Autodesk Inventor part; units mm, degrees
(part 2 of 2)
  arc A179 (-8.5428, 20.014) -> (-8.1409, 20.1954) centre (-9.6846, 23.0787) ccw
  arc A180 (-9.5743, 19.8012) -> (-8.5428, 20.014) centre (-9.7473, 23.247) ccw
  arc A181 (-10.6109, 19.9132) -> (-9.5743, 19.8012) centre (-9.7407, 23.1144) ccw
  arc A182 (-11.5656, 20.3424) -> (-10.6109, 19.9132) centre (-9.7333, 23.1418) ccw
  arc A183 (-12.3588, 21.0513) -> (-11.5656, 20.3424) centre (-9.6135, 23.3247) ccw
  line L45 (-12.3588, 21.0513) -> (-12.436, 21.1445)
  line L46 (-12.436, 21.1445) -> (-12.8142, 20.787)
  line L47 (-12.8142, 20.787) -> (-13.1923, 20.4294)
  line L48 (-13.1923, 20.4294) -> (-13.1528, 20.3728)
  arc A184 (-13.1528, 20.3728) -> (-13.1252, 20.3384) centre (-12.8824, 20.5615) ccw
  arc A185 (-13.1252, 20.3384) -> (-13.0498, 20.2573) centre (-6.3279, 26.584) ccw
  arc A186 (-13.0498, 20.2573) -> (-12.9584, 20.1617) centre (-6.8687, 26.075) ccw
  arc A187 (-12.9584, 20.1617) -> (-12.8577, 20.0592) centre (-4.4477, 28.4259) ccw
  arc A188 (-12.8577, 20.0592) -> (-12.5717, 19.7931) centre (-9.2726, 23.6258) ccw
  arc A189 (-12.5717, 19.7931) -> (-12.2821, 19.5663) centre (-9.9736, 22.8114) ccw
  arc A190 (-12.2821, 19.5663) -> (-11.9733, 19.3675) centre (-9.9819, 22.7997) ccw
  arc A191 (-11.9733, 19.3675) -> (-11.6297, 19.1857) centre (-9.4749, 23.6737) ccw
  arc A192 (-11.6297, 19.1857) -> (-11.2883, 19.0399) centre (-9.8103, 22.9749) ccw
  arc A193 (-11.2883, 19.0399) -> (-10.9284, 18.9216) centre (-9.686, 23.306) ccw
  arc A194 (-10.9284, 18.9216) -> (-10.5594, 18.8334) centre (-9.6828, 23.3174) ccw
  arc A195 (-10.5594, 18.8334) -> (-10.1908, 18.7779) centre (-9.742, 23.0144) ccw
  arc A196 (-10.1908, 18.7779) -> (-9.9934, 18.7649) centre (-9.929, 21.2498) ccw
  arc A197 (-9.9934, 18.7649) -> (-9.7075, 18.7614) centre (-9.7234, 29.1694) ccw
  arc A198 (-9.7075, 18.7614) -> (-9.4242, 18.7657) centre (-9.7237, 29.3221) ccw
  arc A199 (-9.4242, 18.7657) -> (-9.2413, 18.7794) centre (-9.4803, 20.7415) ccw
  arc A200 (-9.5434, 20.4503) -> (-9.0552, 20.5352) centre (-9.8712, 23.7792) ccw
  arc A201 (-9.0552, 20.5352) -> (-8.6122, 20.6889) centre (-9.7096, 23.1369) ccw
  arc A202 (-8.6122, 20.6889) -> (-8.2116, 20.9135) centre (-9.6623, 23.0313) ccw
  arc A203 (-8.2116, 20.9135) -> (-7.8493, 21.2097) centre (-9.7746, 23.1952) ccw
  arc A204 (-7.8493, 21.2097) -> (-7.7329, 21.3272) centre (-10.6671, 24.1156) ccw
  arc A205 (-7.7329, 21.3272) -> (-7.622, 21.4489) centre (-10.618, 24.069) ccw
  arc A206 (-7.622, 21.4489) -> (-7.5253, 21.5617) centre (-13.3375, 26.4473) ccw
  arc A207 (-7.5253, 21.5617) -> (-7.5138, 21.5934) centre (-7.563, 21.5934) ccw
  arc A208 (-7.5138, 21.5934) -> (-7.5197, 21.607) centre (-7.5325, 21.5934) ccw
  arc A209 (-7.5197, 21.607) -> (-7.884, 21.95) centre (-910.3811, -936.9121) ccw
  arc A210 (-7.884, 21.95) -> (-8.2435, 22.2882) centre (-469.987, -469.0133) ccw
  arc A211 (-8.2435, 22.2882) -> (-8.2689, 22.3041) centre (-8.2969, 22.2313) ccw
  arc A212 (-8.2689, 22.3041) -> (-8.2777, 22.3021) centre (-8.2718, 22.2966) ccw
  arc A213 (-8.2777, 22.3021) -> (-8.3041, 22.2731) centre (-7.5009, 21.5676) ccw
  arc A214 (-8.3041, 22.2731) -> (-8.3348, 22.236) centre (-7.7116, 21.7527) ccw
  arc A215 (-8.3348, 22.236) -> (-8.3684, 22.1908) centre (-7.1758, 21.3372) ccw
  arc A216 (-8.5704, 21.9586) -> (-8.3684, 22.1908) centre (-9.6953, 23.1405) ccw
  arc A217 (-8.8146, 21.7653) -> (-8.5704, 21.9586) centre (-9.7506, 23.1987) ccw
  arc A218 (-9.0914, 21.6184) -> (-8.8146, 21.7653) centre (-9.7618, 23.2158) ccw
  arc A219 (-9.3897, 21.524) -> (-9.0914, 21.6184) centre (-9.7586, 23.2082) ccw
  arc A220 (-9.5647, 21.5009) -> (-9.3897, 21.524) centre (-9.6138, 22.5471) ccw
  arc A221 (-9.7914, 21.4994) -> (-9.5647, 21.5009) centre (-9.6959, 24.2957) ccw
  arc A222 (-10.0176, 21.5163) -> (-9.7914, 21.4994) centre (-9.6958, 24.2978) ccw
  arc A223 (-10.1914, 21.5513) -> (-10.0176, 21.5163) centre (-9.8956, 22.5709) ccw
  arc A224 (-10.4567, 21.6554) -> (-10.1914, 21.5513) centre (-9.7563, 23.051) ccw
  arc A225 (-10.7116, 21.8099) -> (-10.4567, 21.6554) centre (-9.618, 23.3266) ccw
  arc A226 (-10.938, 22.0024) -> (-10.7116, 21.8099) centre (-9.6252, 23.3166) ccw
  arc A227 (-11.1179, 22.2194) -> (-10.938, 22.0024) centre (-9.8722, 23.0693) ccw
  arc A228 (-11.1179, 22.2194) -> (-11.1427, 22.2537) centre (-11.7714, 21.7735) ccw
  arc A229 (-11.1427, 22.2537) -> (-11.1661, 22.2818) centre (-11.4888, 21.9894) ccw
  arc A230 (-11.1661, 22.2818) -> (-11.1862, 22.3026) centre (-11.4945, 21.9842) ccw
  arc A231 (-11.1862, 22.3026) -> (-11.1949, 22.3043) centre (-11.1919, 22.2966) ccw
  arc A232 (-11.1949, 22.3043) -> (-11.2195, 22.289) centre (-11.1681, 22.2342) ccw
  arc A233 (-11.2195, 22.289) -> (-11.5799, 21.9506) centre (486.2167, -507.9155) ccw
  arc A234 (-11.5799, 21.9506) -> (-11.945, 21.6075) centre (951.9894, -1003.6952) ccw
  arc A235 (-11.945, 21.6075) -> (-11.9507, 21.5943) centre (-11.9326, 21.5943) ccw
  arc A236 (-11.9507, 21.5943) -> (-11.9489, 21.5889) centre (-11.9416, 21.5943) ccw
  arc A237 (-11.9489, 21.5889) -> (-11.923, 21.5541) centre (-5.8217, 26.1081) ccw
  arc A238 (-11.923, 21.5541) -> (-11.8927, 21.5141) centre (-9.796, 23.1417) ccw
  arc A239 (-11.8927, 21.5141) -> (-11.8566, 21.4683) centre (-8.0644, 24.4859) ccw
  arc A240 (-11.8566, 21.4683) -> (-11.6693, 21.2609) centre (-10.1114, 22.857) ccw
  arc A241 (-11.6693, 21.2609) -> (-11.4378, 21.0549) centre (-9.3184, 23.6694) ccw
  arc A242 (-11.4378, 21.0549) -> (-11.1876, 20.8706) centre (-9.3086, 23.6815) ccw
  arc A243 (-11.1876, 20.8706) -> (-10.944, 20.7285) centre (-9.9098, 22.7821) ccw
  arc A244 (-10.944, 20.7285) -> (-10.7872, 20.6592) centre (-10.181, 22.2437) ccw
  arc A245 (-10.7872, 20.6592) -> (-10.5834, 20.5871) centre (-9.2725, 24.618) ccw
  arc A246 (-10.5834, 20.5871) -> (-10.3752, 20.5253) centre (-9.2666, 24.6361) ccw
  arc A247 (-10.3752, 20.5253) -> (-10.2042, 20.4879) centre (-9.9036, 22.274) ccw
  arc A248 (-10.2042, 20.4879) -> (-10.0507, 20.4678) centre (-9.8539, 22.569) ccw
  arc A249 (-10.0507, 20.4678) -> (-9.8548, 20.4531) centre (-9.5485, 25.8313) ccw
  arc A250 (-9.8548, 20.4531) -> (-9.6658, 20.4456) centre (-9.5457, 25.8799) ccw
  arc A251 (-9.6658, 20.4456) -> (-9.5434, 20.4503) centre (-9.6433, 21.4646) ccw
  arc A252 (-9.5151, 22.1652) -> (-9.26, 22.2834) centre (-9.7491, 23.0046) ccw
  arc A253 (-9.26, 22.2834) -> (-9.0536, 22.4774) centre (-9.7633, 23.0256) ccw
  arc A254 (-9.0536, 22.4774) -> (-8.9194, 22.7243) centre (-9.7513, 23.0163) ccw
  arc A255 (-8.9194, 22.7243) -> (-8.8734, 22.9959) centre (-9.6884, 22.9943) ccw
  arc A256 (-8.8734, 22.9959) -> (-8.9614, 23.3705) centre (-9.7212, 22.9942) ccw
  arc A257 (-8.9614, 23.3705) -> (-9.2064, 23.6715) centre (-9.7465, 22.9817) ccw
  arc A258 (-9.2064, 23.6715) -> (-9.5559, 23.8357) centre (-9.7402, 22.9898) ccw
  arc A259 (-9.5559, 23.8357) -> (-9.9363, 23.8281) centre (-9.73, 23.0363) ccw
  arc A260 (-9.9363, 23.8281) -> (-10.1561, 23.7402) centre (-9.6975, 22.9113) ccw
  arc A261 (-10.1561, 23.7402) -> (-10.3382, 23.6031) centre (-9.7607, 23.0257) ccw
  arc A262 (-10.3382, 23.6031) -> (-10.4753, 23.421) centre (-9.7607, 23.0257) ccw
  arc A263 (-10.4753, 23.421) -> (-10.5631, 23.2012) centre (-9.6464, 22.9624) ccw
  arc A264 (-10.5631, 23.2012) -> (-10.5703, 22.8166) centre (-9.767, 22.9938) ccw
  arc A265 (-10.5703, 22.8166) -> (-10.4026, 22.4656) centre (-9.7328, 23.0014) ccw
  arc A266 (-10.4026, 22.4656) -> (-10.0955, 22.2227) centre (-9.7225, 23.0096) ccw
  arc A267 (-10.0955, 22.2227) -> (-9.7141, 22.1398) centre (-9.7268, 23.0004) ccw
  arc A268 (-9.7141, 22.1398) -> (-9.6642, 22.1422) centre (-9.7254, 22.9033) ccw
  arc A269 (-9.6642, 22.1422) -> (-9.6086, 22.1479) centre (-9.7604, 23.3386) ccw
  arc A270 (-9.6086, 22.1479) -> (-9.5557, 22.1559) centre (-9.7521, 23.2734) ccw
  arc A271 (-9.5557, 22.1559) -> (-9.5151, 22.1652) centre (-9.6295, 22.5755) ccw
  line L49 (-31.75, 88.9) -> (-31.75, 1) construction
  line L50 (-31.75, 0) -> (-31.75, 87.9) construction
  circle A272 centre (-51.1412, 94.7932) radius 1.3939
  line L51 (-54.6697, 97.0432) -> (-53.4511, 95.8952)
  line L52 (-58.6222, 100.8483) -> (-57.4051, 99.7017)
  line L53 (-56.6313, 98.9727) -> (-55.4363, 97.8469)
  line L54 (-47.5961, 97.0193) -> (-48.8314, 95.8952)
  line L55 (-43.6602, 100.8483) -> (-44.8199, 99.6308)
  line L56 (-45.5939, 98.9006) -> (-46.8461, 97.8469)
  arc A273 (-48.8314, 95.8952) -> (-53.4511, 95.8952) centre (-51.1412, 94.5634) ccw
  arc A274 (-47.5961, 97.0193) -> (-54.6697, 97.0432) centre (-51.1412, 94.5634) ccw
  arc A275 (-45.5939, 98.9006) -> (-56.6313, 98.9727) centre (-51.1412, 94.5634) ccw
  arc A276 (-44.8199, 99.6308) -> (-57.4051, 99.7017) centre (-51.1412, 94.5634) ccw
  arc A277 (-43.6602, 100.8483) -> (-58.6222, 100.8483) centre (-51.1412, 94.5634) ccw
  arc A278 (-46.8461, 97.8469) -> (-55.4363, 97.8469) centre (-51.1412, 94.5634) ccw
  circle A279 centre (-40.9176, 68.0261) radius 1.3939
  line L57 (-44.446, 70.2761) -> (-43.2274, 69.1281)
  line L58 (-48.3986, 74.0812) -> (-47.1814, 72.9346)
  line L59 (-46.4077, 72.2056) -> (-45.2126, 71.0798)
  line L60 (-37.3725, 70.2522) -> (-38.6077, 69.1281)
  line L61 (-35.3703, 72.1335) -> (-36.6225, 71.0798)
  line L62 (-33.4365, 74.0812) -> (-34.5962, 72.8637)
  arc A280 (-38.6077, 69.1281) -> (-43.2274, 69.1281) centre (-40.9176, 67.7964) ccw
  arc A281 (-37.3725, 70.2522) -> (-44.446, 70.2761) centre (-40.9176, 67.7964) ccw
  arc A282 (-35.3703, 72.1335) -> (-46.4077, 72.2056) centre (-40.9176, 67.7964) ccw
  arc A283 (-34.5962, 72.8637) -> (-47.1814, 72.9346) centre (-40.9176, 67.7964) ccw
  arc A284 (-33.4365, 74.0812) -> (-48.3986, 74.0812) centre (-40.9176, 67.7964) ccw
  arc A285 (-36.6225, 71.0798) -> (-45.2126, 71.0798) centre (-40.9176, 67.7964) ccw
  circle A286 centre (-22.651, 67.9533) radius 1.3939
  line L63 (-26.1795, 70.2033) -> (-24.9609, 69.0553)
  line L64 (-30.132, 74.0084) -> (-28.9149, 72.8617)
  line L65 (-28.1412, 72.1328) -> (-26.9461, 71.007)
  line L66 (-19.106, 70.1794) -> (-20.3412, 69.0553)
  line L67 (-17.1038, 72.0606) -> (-18.356, 71.007)
  line L68 (-15.17, 74.0084) -> (-16.3297, 72.7909)
  arc A287 (-20.3412, 69.0553) -> (-24.9609, 69.0553) centre (-22.651, 67.7235) ccw
  arc A288 (-19.106, 70.1794) -> (-26.1795, 70.2033) centre (-22.651, 67.7235) ccw
  arc A289 (-17.1038, 72.0606) -> (-28.1412, 72.1328) centre (-22.651, 67.7235) ccw
  arc A290 (-16.3297, 72.7909) -> (-28.9149, 72.8617) centre (-22.651, 67.7235) ccw
  arc A291 (-15.17, 74.0084) -> (-30.132, 74.0084) centre (-22.651, 67.7235) ccw
  arc A292 (-18.356, 71.007) -> (-26.9461, 71.007) centre (-22.651, 67.7235) ccw
  circle A293 centre (-40.9176, 20.8739) radius 1.3939
  line L69 (-37.3725, 18.6478) -> (-38.6077, 19.7719)
  arc A294 (-43.2274, 19.7719) -> (-38.6077, 19.7719) centre (-40.9176, 21.1036) ccw
  line L70 (-44.446, 18.6239) -> (-43.2274, 19.7719)
  arc A295 (-44.446, 18.6239) -> (-37.3725, 18.6478) centre (-40.9176, 21.1036) ccw
  line L71 (-33.4365, 14.8188) -> (-34.5962, 16.0363)
  arc A296 (-45.2126, 17.8202) -> (-36.6225, 17.8202) centre (-40.9176, 21.1036) ccw
  arc A297 (-46.4077, 16.6944) -> (-35.3703, 16.7665) centre (-40.9176, 21.1036) ccw
  arc A298 (-47.1814, 15.9654) -> (-34.5962, 16.0363) centre (-40.9176, 21.1036) ccw
  arc A299 (-48.3986, 14.8188) -> (-33.4365, 14.8188) centre (-40.9176, 21.1036) ccw
  line L72 (-35.3703, 16.7665) -> (-36.6225, 17.8202)
  line L73 (-48.3986, 14.8188) -> (-47.1814, 15.9654)
  line L74 (-46.4077, 16.6944) -> (-45.2126, 17.8202)
  circle A300 centre (-22.651, 20.9467) radius 1.3939
  line L75 (-19.106, 18.7206) -> (-20.3412, 19.8447)
  arc A301 (-24.9609, 19.8447) -> (-20.3412, 19.8447) centre (-22.651, 21.1765) ccw
  line L76 (-26.1795, 18.6967) -> (-24.9609, 19.8447)
  arc A302 (-26.1795, 18.6967) -> (-19.106, 18.7206) centre (-22.651, 21.1765) ccw
  line L77 (-15.17, 14.8916) -> (-16.3297, 16.1091)
  arc A303 (-26.9461, 17.893) -> (-18.356, 17.893) centre (-22.651, 21.1765) ccw
  arc A304 (-28.1412, 16.7672) -> (-17.1038, 16.8394) centre (-22.651, 21.1765) ccw
  arc A305 (-28.9149, 16.0383) -> (-16.3297, 16.1091) centre (-22.651, 21.1765) ccw
  arc A306 (-30.132, 14.8916) -> (-15.17, 14.8916) centre (-22.651, 21.1765) ccw
  line L78 (-17.1038, 16.8394) -> (-18.356, 17.893)
  line L79 (-30.132, 14.8916) -> (-28.9149, 16.0383)
  line L80 (-28.1412, 16.7672) -> (-26.9461, 17.893)
  line L81 (-62.5, 44.45) -> (-1, 44.45) construction
  circle A307 centre (-48.3683, 40.8951) radius 1.3939
  line L82 (-51.8968, 43.1451) -> (-50.6782, 41.9971)
  line L83 (-55.8493, 46.9502) -> (-54.6322, 45.8036)
  line L84 (-53.8584, 45.0746) -> (-52.6634, 43.9488)
  line L85 (-44.8232, 43.1213) -> (-46.0585, 41.9971)
  line L86 (-42.821, 45.0025) -> (-44.0732, 43.9488)
  line L87 (-40.8873, 46.9502) -> (-42.047, 45.7328)
  arc A308 (-46.0585, 41.9971) -> (-50.6782, 41.9971) centre (-48.3683, 40.6654) ccw
  arc A309 (-44.8232, 43.1213) -> (-51.8968, 43.1451) centre (-48.3683, 40.6654) ccw
  arc A310 (-42.821, 45.0025) -> (-53.8584, 45.0746) centre (-48.3683, 40.6654) ccw
  arc A311 (-42.047, 45.7328) -> (-54.6322, 45.8036) centre (-48.3683, 40.6654) ccw
  arc A312 (-40.8873, 46.9502) -> (-55.8493, 46.9502) centre (-48.3683, 40.6654) ccw
  arc A313 (-44.0732, 43.9488) -> (-52.6634, 43.9488) centre (-48.3683, 40.6654) ccw
  line L88 (-40.9176, 72.907) -> (-15.0551, 45.776) construction
  line L89 (-40.9176, 44.45) -> (-22.651, 72.8342) construction
  circle A314 centre (-31.7554, 53.8061) radius 1.3939
  line L90 (-35.2839, 56.0561) -> (-34.0653, 54.9081)
  line L91 (-39.2364, 59.8611) -> (-38.0193, 58.7145)
  line L92 (-37.2455, 57.9856) -> (-36.0505, 56.8598)
  line L93 (-28.2104, 56.0322) -> (-29.4456, 54.9081)
  line L94 (-26.2081, 57.9134) -> (-27.4604, 56.8598)
  line L95 (-24.2744, 59.8611) -> (-25.4341, 58.6437)
  arc A315 (-29.4456, 54.9081) -> (-34.0653, 54.9081) centre (-31.7554, 53.5763) ccw
  arc A316 (-28.2104, 56.0322) -> (-35.2839, 56.0561) centre (-31.7554, 53.5763) ccw
  arc A317 (-26.2081, 57.9134) -> (-37.2455, 57.9856) centre (-31.7554, 53.5763) ccw
  arc A318 (-25.4341, 58.6437) -> (-38.0193, 58.7145) centre (-31.7554, 53.5763) ccw
  arc A319 (-24.2744, 59.8611) -> (-39.2364, 59.8611) centre (-31.7554, 53.5763) ccw
  arc A320 (-27.4604, 56.8598) -> (-36.0505, 56.8598) centre (-31.7554, 53.5763) ccw
  line L96 (-35.2839, 32.8439) -> (-34.0653, 33.9919)
  line L97 (-37.2455, 30.9144) -> (-36.0505, 32.0402)
  line L98 (-39.2364, 29.0389) -> (-38.0193, 30.1855)
  circle A321 centre (-31.7554, 35.0939) radius 1.3939
  arc A322 (-34.0653, 33.9919) -> (-29.4456, 33.9919) centre (-31.7554, 35.3237) ccw
  arc A323 (-35.2839, 32.8439) -> (-28.2104, 32.8678) centre (-31.7554, 35.3237) ccw
  arc A324 (-36.0505, 32.0402) -> (-27.4604, 32.0402) centre (-31.7554, 35.3237) ccw
  arc A325 (-37.2455, 30.9144) -> (-26.2081, 30.9866) centre (-31.7554, 35.3237) ccw
  arc A326 (-39.2364, 29.0389) -> (-24.2744, 29.0389) centre (-31.7554, 35.3237) ccw
  arc A327 (-38.0193, 30.1855) -> (-25.4341, 30.2563) centre (-31.7554, 35.3237) ccw
  line L99 (-28.2104, 32.8678) -> (-29.4456, 33.9919)
  line L100 (-26.2081, 30.9866) -> (-27.4604, 32.0402)
  line L101 (-24.2744, 29.0389) -> (-25.4341, 30.2563)
  line L102 (-11.6032, 43.1451) -> (-12.8218, 41.9971)
  line L103 (-9.6416, 45.0746) -> (-10.8366, 43.9488)
  line L104 (-7.6507, 46.9502) -> (-8.8678, 45.8036)
  arc A328 (-12.8218, 41.9971) -> (-17.4415, 41.9971) centre (-15.1317, 40.6654) ccw
  arc A329 (-7.6507, 46.9502) -> (-22.6127, 46.9502) centre (-15.1317, 40.6654) ccw
  arc A330 (-8.8678, 45.8036) -> (-21.453, 45.7328) centre (-15.1317, 40.6654) ccw
  arc A331 (-9.6416, 45.0746) -> (-20.679, 45.0025) centre (-15.1317, 40.6654) ccw
  arc A332 (-10.8366, 43.9488) -> (-19.4268, 43.9488) centre (-15.1317, 40.6654) ccw
  arc A333 (-11.6032, 43.1451) -> (-18.6768, 43.1213) centre (-15.1317, 40.6654) ccw
  circle A334 centre (-15.1317, 40.8951) radius 1.3939
  line L105 (-18.6768, 43.1213) -> (-17.4415, 41.9971)
  line L106 (-20.679, 45.0025) -> (-19.4268, 43.9488)
  line L107 (-22.6127, 46.9502) -> (-21.453, 45.7328)
  line L108 (-35.2402, 43.1451) -> (-34.0216, 41.9971)
  line L109 (-37.2018, 45.0746) -> (-36.0068, 43.9488)
  line L110 (-39.1927, 46.9502) -> (-37.9756, 45.8036)
  arc A335 (-29.4019, 41.9971) -> (-34.0216, 41.9971) centre (-31.7117, 40.6654) ccw
  arc A336 (-24.2307, 46.9502) -> (-39.1927, 46.9502) centre (-31.7117, 40.6654) ccw
  arc A337 (-25.3904, 45.7328) -> (-37.9756, 45.8036) centre (-31.7117, 40.6654) ccw
  arc A338 (-26.1644, 45.0025) -> (-37.2018, 45.0746) centre (-31.7117, 40.6654) ccw
  arc A339 (-27.4166, 43.9488) -> (-36.0068, 43.9488) centre (-31.7117, 40.6654) ccw
  arc A340 (-28.1666, 43.1213) -> (-35.2402, 43.1451) centre (-31.7117, 40.6654) ccw
  circle A341 centre (-31.7117, 40.8951) radius 1.3939
  line L111 (-28.1666, 43.1213) -> (-29.4019, 41.9971)
  line L112 (-26.1644, 45.0025) -> (-27.4166, 43.9488)
  line L113 (-24.2307, 46.9502) -> (-25.3904, 45.7328)
  spline S0 degree 2 poles (-57.0989, 82.3254) (-57.0989, 83.1076) (-56.5885, 84.4085) (-56.1439, 84.8778) knots 0 0 0 1 2 2 2
  spline S1 degree 2 poles (-56.1439, 84.8778) (-55.724, 85.3306) (-54.4972, 85.8328) (-53.8714, 85.8328) knots 0 0 0 1 2 2 2
  spline S2 degree 2 poles (-53.8714, 85.8328) (-53.1716, 85.8328) (-52.0354, 85.3635) (-51.6155, 84.9189) knots 0 0 0 1 2 2 2
  spline S3 degree 2 poles (-51.6155, 84.9189) (-51.0886, 84.3591) (-50.5122, 82.5477) (-50.5122, 81.1563) knots 0 0 0 1 2 2 2
  spline S4 degree 2 poles (-50.5122, 81.1563) (-50.5122, 79.8966) (-51.0803, 77.6406) (-51.632, 76.8914) knots 0 0 0 1 2 2 2
  spline S5 degree 2 poles (-51.632, 76.8914) (-52.2165, 76.101) (-53.8632, 75.2694) (-55.0653, 75.2694) knots 0 0 0 1 2 2 2
  spline S6 degree 2 poles (-55.0653, 75.2694) (-55.337, 75.2694) (-55.9545, 75.327) (-56.218, 75.4094) knots 0 0 0 1 2 2 2
  line L114 (-56.218, 75.4094) -> (-56.218, 76.7185)
  line L115 (-56.218, 76.7185) -> (-56.1521, 76.7185)
  spline S7 degree 2 poles (-56.1521, 76.7185) (-55.9792, 76.6197) (-55.2546, 76.4468) (-54.8841, 76.4468) knots 0 0 0 1 2 2 2
  spline S8 degree 2 poles (-54.8841, 76.4468) (-53.5503, 76.4468) (-52.0272, 78.2087) (-51.9201, 79.8389) knots 0 0 0 1 2 2 2
  spline S9 degree 2 poles (-51.9201, 79.8389) (-52.4635, 79.4684) (-53.4515, 79.1309) (-54.0361, 79.1309) knots 0 0 0 1 2 2 2
  spline S10 degree 2 poles (-54.0361, 79.1309) (-54.596, 79.1309) (-55.5264, 79.3779) (-55.9957, 79.7319) knots 0 0 0 1 2 2 2
  spline S11 degree 2 poles (-55.9957, 79.7319) (-56.5391, 80.1518) (-57.0989, 81.428) (-57.0989, 82.3254) knots 0 0 0 1 2 2 2
  spline S12 degree 2 poles (-51.8872, 81.4609) (-51.8872, 82.4901) (-52.2659, 83.7909) (-52.6035, 84.145) knots 0 0 0 1 2 2 2
  spline S13 degree 2 poles (-52.6035, 84.145) (-52.8999, 84.4743) (-53.5174, 84.7213) (-53.8797, 84.7213) knots 0 0 0 1 2 2 2
  spline S14 degree 2 poles (-53.8797, 84.7213) (-54.7195, 84.7213) (-55.7157, 83.5192) (-55.7157, 82.383) knots 0 0 0 1 2 2 2
  spline S15 degree 2 poles (-55.7157, 82.383) (-55.7157, 81.7408) (-55.3864, 80.9093) (-55.0241, 80.6129) knots 0 0 0 1 2 2 2
  spline S16 degree 2 poles (-55.0241, 80.6129) (-54.7606, 80.3988) (-54.1102, 80.2588) (-53.7315, 80.2588) knots 0 0 0 1 2 2 2
  spline S17 degree 2 poles (-53.7315, 80.2588) (-53.2951, 80.2588) (-52.2906, 80.5635) (-51.9119, 80.8187) knots 0 0 0 1 2 2 2
  spline S18 degree 2 poles (-51.9119, 80.8187) (-51.9037, 80.9175) (-51.8872, 81.2551) (-51.8872, 81.4609) knots 0 0 0 1 2 2 2
  spline S19 degree 2 poles (-6.4011, 6.9192) (-6.4011, 6.137) (-6.9115, 4.8361) (-7.3561, 4.3668) knots 0 0 0 1 2 2 2
  spline S20 degree 2 poles (-7.3561, 4.3668) (-7.776, 3.914) (-9.0028, 3.4117) (-9.6286, 3.4117) knots 0 0 0 1 2 2 2
  spline S21 degree 2 poles (-9.6286, 3.4117) (-10.3284, 3.4117) (-11.4646, 3.881) (-11.8845, 4.3257) knots 0 0 0 1 2 2 2
  spline S22 degree 2 poles (-11.8845, 4.3257) (-12.4114, 4.8855) (-12.9878, 6.6969) (-12.9878, 8.0883) knots 0 0 0 1 2 2 2
  spline S23 degree 2 poles (-12.9878, 8.0883) (-12.9878, 9.348) (-12.4197, 11.604) (-11.868, 12.3532) knots 0 0 0 1 2 2 2
  spline S24 degree 2 poles (-11.868, 12.3532) (-11.2835, 13.1436) (-9.6368, 13.9752) (-8.4347, 13.9752) knots 0 0 0 1 2 2 2
  spline S25 degree 2 poles (-8.4347, 13.9752) (-8.163, 13.9752) (-7.5455, 13.9175) (-7.282, 13.8352) knots 0 0 0 1 2 2 2
  line L116 (-7.282, 13.8352) -> (-7.282, 12.5261)
  line L117 (-7.282, 12.5261) -> (-7.3479, 12.5261)
  spline S26 degree 2 poles (-7.3479, 12.5261) (-7.5208, 12.6249) (-8.2454, 12.7978) (-8.6159, 12.7978) knots 0 0 0 1 2 2 2
  spline S27 degree 2 poles (-8.6159, 12.7978) (-9.9497, 12.7978) (-11.4728, 11.0359) (-11.5799, 9.4057) knots 0 0 0 1 2 2 2
  spline S28 degree 2 poles (-11.5799, 9.4057) (-11.0365, 9.7762) (-10.0485, 10.1137) (-9.4639, 10.1137) knots 0 0 0 1 2 2 2
  spline S29 degree 2 poles (-9.4639, 10.1137) (-8.904, 10.1137) (-7.9736, 9.8667) (-7.5043, 9.5127) knots 0 0 0 1 2 2 2
  spline S30 degree 2 poles (-7.5043, 9.5127) (-6.9609, 9.0928) (-6.4011, 7.8166) (-6.4011, 6.9192) knots 0 0 0 1 2 2 2
  spline S31 degree 2 poles (-11.6128, 7.7837) (-11.6128, 6.7545) (-11.2341, 5.4536) (-10.8965, 5.0996) knots 0 0 0 1 2 2 2
  spline S32 degree 2 poles (-10.8965, 5.0996) (-10.6001, 4.7703) (-9.9826, 4.5233) (-9.6203, 4.5233) knots 0 0 0 1 2 2 2
  spline S33 degree 2 poles (-9.6203, 4.5233) (-8.7805, 4.5233) (-7.7843, 5.7253) (-7.7843, 6.8615) knots 0 0 0 1 2 2 2
  spline S34 degree 2 poles (-7.7843, 6.8615) (-7.7843, 7.5037) (-8.1136, 8.3353) (-8.4759, 8.6317) knots 0 0 0 1 2 2 2
  spline S35 degree 2 poles (-8.4759, 8.6317) (-8.7394, 8.8458) (-9.3898, 8.9857) (-9.7685, 8.9857) knots 0 0 0 1 2 2 2
  spline S36 degree 2 poles (-9.7685, 8.9857) (-10.2049, 8.9857) (-11.2094, 8.6811) (-11.5881, 8.4259) knots 0 0 0 1 2 2 2
  spline S37 degree 2 poles (-11.5881, 8.4259) (-11.5963, 8.3271) (-11.6128, 7.9895) (-11.6128, 7.7837) knots 0 0 0 1 2 2 2
  spline S38 degree 2 poles (-57.0989, 82.3254) (-57.0989, 83.1076) (-56.5885, 84.4085) (-56.1439, 84.8778) knots 0 0 0 1 2 2 2
  spline S39 degree 2 poles (-56.1439, 84.8778) (-55.724, 85.3306) (-54.4972, 85.8328) (-53.8714, 85.8328) knots 0 0 0 1 2 2 2
  spline S40 degree 2 poles (-53.8714, 85.8328) (-53.1716, 85.8328) (-52.0354, 85.3635) (-51.6155, 84.9189) knots 0 0 0 1 2 2 2
  spline S41 degree 2 poles (-51.6155, 84.9189) (-51.0886, 84.3591) (-50.5122, 82.5477) (-50.5122, 81.1563) knots 0 0 0 1 2 2 2
  spline S42 degree 2 poles (-50.5122, 81.1563) (-50.5122, 79.8966) (-51.0803, 77.6406) (-51.632, 76.8914) knots 0 0 0 1 2 2 2
  spline S43 degree 2 poles (-51.632, 76.8914) (-52.2165, 76.101) (-53.8632, 75.2694) (-55.0653, 75.2694) knots 0 0 0 1 2 2 2
  spline S44 degree 2 poles (-55.0653, 75.2694) (-55.337, 75.2694) (-55.9545, 75.327) (-56.218, 75.4094) knots 0 0 0 1 2 2 2
  line L118 (-56.218, 75.4094) -> (-56.218, 76.7185)
  line L119 (-56.218, 76.7185) -> (-56.1521, 76.7185)
  spline S45 degree 2 poles (-56.1521, 76.7185) (-55.9792, 76.6197) (-55.2546, 76.4468) (-54.8841, 76.4468) knots 0 0 0 1 2 2 2
  spline S46 degree 2 poles (-54.8841, 76.4468) (-53.5503, 76.4468) (-52.0272, 78.2087) (-51.9201, 79.8389) knots 0 0 0 1 2 2 2
  spline S47 degree 2 poles (-51.9201, 79.8389) (-52.4635, 79.4684) (-53.4515, 79.1309) (-54.0361, 79.1309) knots 0 0 0 1 2 2 2
  spline S48 degree 2 poles (-54.0361, 79.1309) (-54.596, 79.1309) (-55.5264, 79.3779) (-55.9957, 79.7319) knots 0 0 0 1 2 2 2
  spline S49 degree 2 poles (-55.9957, 79.7319) (-56.5391, 80.1518) (-57.0989, 81.428) (-57.0989, 82.3254) knots 0 0 0 1 2 2 2
  spline S50 degree 2 poles (-51.8872, 81.4609) (-51.8872, 82.4901) (-52.2659, 83.7909) (-52.6035, 84.145) knots 0 0 0 1 2 2 2
  spline S51 degree 2 poles (-52.6035, 84.145) (-52.8999, 84.4743) (-53.5174, 84.7213) (-53.8797, 84.7213) knots 0 0 0 1 2 2 2
  spline S52 degree 2 poles (-53.8797, 84.7213) (-54.7195, 84.7213) (-55.7157, 83.5192) (-55.7157, 82.383) knots 0 0 0 1 2 2 2
  spline S53 degree 2 poles (-55.7157, 82.383) (-55.7157, 81.7408) (-55.3864, 80.9093) (-55.0241, 80.6129) knots 0 0 0 1 2 2 2
  spline S54 degree 2 poles (-55.0241, 80.6129) (-54.7606, 80.3988) (-54.1102, 80.2588) (-53.7315, 80.2588) knots 0 0 0 1 2 2 2
  spline S55 degree 2 poles (-53.7315, 80.2588) (-53.2951, 80.2588) (-52.2906, 80.5635) (-51.9119, 80.8187) knots 0 0 0 1 2 2 2
  spline S56 degree 2 poles (-51.9119, 80.8187) (-51.9037, 80.9175) (-51.8872, 81.2551) (-51.8872, 81.4609) knots 0 0 0 1 2 2 2
  spline S57 degree 2 poles (-6.4011, 6.9192) (-6.4011, 6.137) (-6.9115, 4.8361) (-7.3561, 4.3668) knots 0 0 0 1 2 2 2
  spline S58 degree 2 poles (-7.3561, 4.3668) (-7.776, 3.914) (-9.0028, 3.4117) (-9.6286, 3.4117) knots 0 0 0 1 2 2 2
  spline S59 degree 2 poles (-9.6286, 3.4117) (-10.3284, 3.4117) (-11.4646, 3.881) (-11.8845, 4.3257) knots 0 0 0 1 2 2 2
  spline S60 degree 2 poles (-11.8845, 4.3257) (-12.4114, 4.8855) (-12.9878, 6.6969) (-12.9878, 8.0883) knots 0 0 0 1 2 2 2
  spline S61 degree 2 poles (-12.9878, 8.0883) (-12.9878, 9.348) (-12.4197, 11.604) (-11.868, 12.3532) knots 0 0 0 1 2 2 2
  spline S62 degree 2 poles (-11.868, 12.3532) (-11.2835, 13.1436) (-9.6368, 13.9752) (-8.4347, 13.9752) knots 0 0 0 1 2 2 2
  spline S63 degree 2 poles (-8.4347, 13.9752) (-8.163, 13.9752) (-7.5455, 13.9175) (-7.282, 13.8352) knots 0 0 0 1 2 2 2
  line L120 (-7.282, 13.8352) -> (-7.282, 12.5261)
  line L121 (-7.282, 12.5261) -> (-7.3479, 12.5261)
  spline S64 degree 2 poles (-7.3479, 12.5261) (-7.5208, 12.6249) (-8.2454, 12.7978) (-8.6159, 12.7978) knots 0 0 0 1 2 2 2
  spline S65 degree 2 poles (-8.6159, 12.7978) (-9.9497, 12.7978) (-11.4728, 11.0359) (-11.5799, 9.4057) knots 0 0 0 1 2 2 2
  spline S66 degree 2 poles (-11.5799, 9.4057) (-11.0365, 9.7762) (-10.0485, 10.1137) (-9.4639, 10.1137) knots 0 0 0 1 2 2 2
  spline S67 degree 2 poles (-9.4639, 10.1137) (-8.904, 10.1137) (-7.9736, 9.8667) (-7.5043, 9.5127) knots 0 0 0 1 2 2 2
  spline S68 degree 2 poles (-7.5043, 9.5127) (-6.9609, 9.0928) (-6.4011, 7.8166) (-6.4011, 6.9192) knots 0 0 0 1 2 2 2
  spline S69 degree 2 poles (-11.6128, 7.7837) (-11.6128, 6.7545) (-11.2341, 5.4536) (-10.8965, 5.0996) knots 0 0 0 1 2 2 2
  spline S70 degree 2 poles (-10.8965, 5.0996) (-10.6001, 4.7703) (-9.9826, 4.5233) (-9.6203, 4.5233) knots 0 0 0 1 2 2 2
  spline S71 degree 2 poles (-9.6203, 4.5233) (-8.7805, 4.5233) (-7.7843, 5.7253) (-7.7843, 6.8615) knots 0 0 0 1 2 2 2
  spline S72 degree 2 poles (-7.7843, 6.8615) (-7.7843, 7.5037) (-8.1136, 8.3353) (-8.4759, 8.6317) knots 0 0 0 1 2 2 2
  spline S73 degree 2 poles (-8.4759, 8.6317) (-8.7394, 8.8458) (-9.3898, 8.9857) (-9.7685, 8.9857) knots 0 0 0 1 2 2 2
  spline S74 degree 2 poles (-9.7685, 8.9857) (-10.2049, 8.9857) (-11.2094, 8.6811) (-11.5881, 8.4259) knots 0 0 0 1 2 2 2
  spline S75 degree 2 poles (-11.5881, 8.4259) (-11.5963, 8.3271) (-11.6128, 7.9895) (-11.6128, 7.7837) knots 0 0 0 1 2 2 2
  point P0 (-53.7479, 68.8958)
  point P1 (-53.7479, 68.8958)
  point P2 (-9.7521, 20.0042)
  point P3 (-9.7521, 20.0042)
  point P4 (-10.5703, 22.8165)
  point P5 (-10.4026, 22.4657)
  point P6 (-10.0955, 22.2226)
  point P7 (-9.7141, 22.1398)
  point P8 (-9.6642, 22.1422)
  point P9 (-9.6086, 22.1479)
  point P10 (-9.5557, 22.1559)
  point P11 (-9.5151, 22.1652)
  point P12 (-9.2599, 22.2834)
  point P13 (-9.0536, 22.4773)
  point P14 (-8.9194, 22.7243)
  point P15 (-8.8734, 22.9959)
  point P16 (-8.9615, 23.3705)
  point P17 (-9.2064, 23.6715)
  point P18 (-9.5559, 23.8357)
  point P19 (-9.9363, 23.8281)
  point P20 (-10.1561, 23.7402)
  point P21 (-10.3382, 23.6031)
  point P22 (-10.4753, 23.421)
  point P23 (-10.5631, 23.2012)
  point P24 (-11.1179, 22.2194)
  point P25 (-11.1427, 22.2537)
  point P26 (-11.1661, 22.2818)
  point P27 (-11.1862, 22.3026)
  point P28 (-11.1949, 22.3043)
  point P29 (-11.2195, 22.289)
  point P30 (-11.5796, 21.9509)
  point P31 (-11.945, 21.6075)
  point P32 (-11.9503, 21.5909)
  point P33 (-11.923, 21.5541)
  point P34 (-11.8927, 21.5141)
  point P35 (-11.8566, 21.4683)
  point P36 (-11.6693, 21.2609)
  point P37 (-11.4387, 21.0557)
  point P38 (-11.1876, 20.8705)
  point P39 (-10.944, 20.7285)
  point P40 (-10.7872, 20.6592)
  point P41 (-10.5831, 20.587)
  point P42 (-10.3752, 20.5253)
  point P43 (-10.2042, 20.4879)
  point P44 (-10.0507, 20.4678)
  point P45 (-9.8557, 20.4531)
  point P46 (-9.6658, 20.4456)
  point P47 (-9.5434, 20.4503)
  point P48 (-9.0551, 20.5352)
  point P49 (-8.6122, 20.6889)
  point P50 (-8.2116, 20.9135)
  point P51 (-7.8493, 21.2097)
  point P52 (-7.7331, 21.327)
  point P53 (-7.622, 21.4489)
  point P54 (-7.5253, 21.5617)
  point P55 (-7.5138, 21.5934)
  point P56 (-7.5197, 21.607)
  point P57 (-7.8841, 21.9502)
  point P58 (-8.2435, 22.2882)
  point P59 (-8.2689, 22.3041)
  point P60 (-8.2777, 22.3021)
  point P61 (-8.3041, 22.2731)
  point P62 (-8.3348, 22.236)
  point P63 (-8.3684, 22.1908)
  point P64 (-8.5704, 21.9586)
  point P65 (-8.8147, 21.7652)
  point P66 (-9.0914, 21.6184)
  point P67 (-9.3897, 21.524)
  point P68 (-9.5647, 21.5009)
  point P69 (-9.7914, 21.4994)
  point P70 (-10.0176, 21.5163)
  point P71 (-10.1914, 21.5513)
  point P72 (-10.4567, 21.6554)
  point P73 (-10.7116, 21.8099)
  point P74 (-10.938, 22.0024)
  point P75 (-12.3588, 21.0513)
  point P76 (-13.1528, 20.3728)
  point P77 (-13.1252, 20.3384)
  point P78 (-13.0498, 20.2573)
  point P79 (-12.9584, 20.1617)
  point P80 (-12.8577, 20.0592)
  point P81 (-12.5717, 19.7931)
  point P82 (-12.2814, 19.5658)
  point P83 (-11.9733, 19.3675)
  point P84 (-11.6297, 19.1857)
  point P85 (-11.2882, 19.0399)
  point P86 (-10.929, 18.9217)
  point P87 (-10.5594, 18.8334)
  point P88 (-10.1908, 18.7779)
  point P89 (-9.9934, 18.7649)
  point P90 (-9.7081, 18.7614)
  point P91 (-9.4242, 18.7657)
  point P92 (-9.2413, 18.7794)
  point P93 (-8.6534, 18.8889)
  point P94 (-8.0948, 19.0705)
  point P95 (-7.5656, 19.3247)
  point P96 (-7.0606, 19.6529)
  point P97 (-6.8979, 19.7869)
  point P98 (-6.6506, 20.0183)
  point P99 (-6.4104, 20.2542)
  point P100 (-6.311, 20.3732)
  point P101 (-7.1055, 21.0515)
  point P102 (-7.42, 20.7158)
  point P103 (-7.7659, 20.4297)
  point P104 (-8.1412, 20.1952)
  point P105 (-8.5427, 20.014)
  point P106 (-9.5743, 19.8012)
  point P107 (-10.6108, 19.9132)
  point P108 (-11.5656, 20.3424)
  point P109 (-13.5761, 19.866)
  point P110 (-14.3813, 19.2039)
  point P111 (-14.2565, 19.0613)
  point P112 (-14.0091, 18.8162)
  point P113 (-13.7512, 18.5722)
  point P114 (-13.565, 18.4124)
  point P115 (-12.8019, 17.8902)
  point P116 (-11.9796, 17.4914)
  point P117 (-11.104, 17.2199)
  point P118 (-10.1873, 17.0788)
  point P119 (-9.9643, 17.0663)
  point P120 (-9.7126, 17.0625)
  point P121 (-9.4621, 17.0672)
  point P122 (-9.2413, 17.0805)
  point P123 (-8.2838, 17.2366)
  point P124 (-7.377, 17.5341)
  point P125 (-6.5197, 17.9755)
  point P126 (-5.739, 18.5475)
  point P127 (-5.5697, 18.7002)
  point P128 (-5.3759, 18.8891)
  point P129 (-5.1963, 19.0746)
  point P130 (-5.0811, 19.2079)
  point P131 (-5.8882, 19.8662)
  point P132 (-7.1693, 18.8037)
  point P133 (-7.913, 18.4418)
  point P134 (-8.6923, 18.2113)
  point P135 (-9.2058, 18.1331)
  point P136 (-9.7322, 18.107)
  point P137 (-10.2586, 18.1331)
  point P138 (-10.7722, 18.2113)
  point P139 (-11.5515, 18.4415)
  point P140 (-12.2934, 18.8022)
  point P141 (-12.9752, 19.2817)
  point P142 (-53.9849, 66.7348)
  point P143 (-54.2401, 66.6166)
  point P144 (-54.4464, 66.4227)
  point P145 (-54.5806, 66.1757)
  point P146 (-54.6266, 65.9041)
  point P147 (-54.5385, 65.5295)
  point P148 (-54.2936, 65.2285)
  point P149 (-53.9441, 65.0643)
  point P150 (-53.5637, 65.0719)
  point P151 (-53.3439, 65.1598)
  point P152 (-53.1618, 65.2969)
  point P153 (-53.0247, 65.479)
  point P154 (-52.9369, 65.6988)
  point P155 (-52.9297, 66.0835)
  point P156 (-53.0974, 66.4343)
  point P157 (-53.4045, 66.6774)
  point P158 (-53.7859, 66.7602)
  point P159 (-53.8358, 66.7578)
  point P160 (-53.8914, 66.7521)
  point P161 (-53.9443, 66.7441)
  point P162 (-52.3821, 66.6806)
  point P163 (-52.3573, 66.6463)
  point P164 (-52.3339, 66.6182)
  point P165 (-52.3138, 66.5974)
  point P166 (-52.3051, 66.5957)
  point P167 (-52.2805, 66.611)
  point P168 (-51.9204, 66.9491)
  point P169 (-51.555, 67.2925)
  point P170 (-51.5497, 67.3091)
  point P171 (-51.577, 67.3459)
  point P172 (-51.6073, 67.3859)
  point P173 (-51.6434, 67.4317)
  point P174 (-51.8307, 67.6391)
  point P175 (-52.0613, 67.8443)
  point P176 (-52.3124, 68.0295)
  point P177 (-52.556, 68.1715)
  point P178 (-52.7128, 68.2408)
  point P179 (-52.9169, 68.313)
  point P180 (-53.1248, 68.3747)
  point P181 (-53.2958, 68.4121)
  point P182 (-53.4493, 68.4322)
  point P183 (-53.6443, 68.4469)
  point P184 (-53.8342, 68.4544)
  point P185 (-53.9566, 68.4497)
  point P186 (-54.4449, 68.3648)
  point P187 (-54.8878, 68.2111)
  point P188 (-55.2884, 67.9865)
  point P189 (-55.6507, 67.6903)
  point P190 (-55.7669, 67.573)
  point P191 (-55.878, 67.4511)
  point P192 (-55.9747, 67.3383)
  point P193 (-55.9862, 67.3066)
  point P194 (-55.9803, 67.293)
  point P195 (-55.6159, 66.9498)
  point P196 (-55.2565, 66.6118)
  point P197 (-55.2311, 66.5959)
  point P198 (-55.1959, 66.6269)
  point P199 (-55.1652, 66.664)
  dimension "d103" = 8.4153
  dimension "d105" = 0.508
  dimension "d106" = 0.508
  dimension "d111" = 2.9972
  dimension "d112" = -2.9972
  dimension "d142" = 9.1676
  dimension "d143" = 9.1676
  constraints: 664 point on circle, 342 centre point, 204 end point, 88 symmetric about line, 30 concentric, 13 point on line, 5 midpoint, 1 coincident, 1 perpendicular, 32 other
  measures "d103" distance of L12.end L14.start
  measures "d105" distance between parallel lines of L15 L7
  measures "d106" distance between parallel lines of L16 L11
  measures "d111" vertical distance of point (-53.748, 68.896) A129.centre
  measures "d112" vertical distance of point (-9.752, 20.004) A265.centre
  measures "d142" distance from line of L50 L88.start
  measures "d143" horizontal distance of point (-31.75, 87.9) point (-40.918, 44.45)
extrude "Extrusion20" add sketch "Sketch17" along normal blind 0.4 contours A31 A30 A29 A28 A27 A26 A25 A24 A23 A22 A21 A20 L24 L23 L22 L21 A19 A18 A17 A16 A15 A14 A13 A12 A11 A10 A9 A8 L20 L19 L18 L17 A7 A6 A5 A4 A3 A2 A1 A0 | A63 A62 A61 A60 A59 A58 A57 A56 A55 A54 A53 A52 A51 A50 A49 A48 L32 L31 L30 L29 A47 A46 A45 A44 A43 A42 A41 A40 L28 L27 L26 L25 A39 A38 A37 A36 A35 A34 A33 A32 | A115 A114 A113 A112 A111 A110 A109 A108 A107 A106 A105 A104 A103 A102 A101 A100 A99 A98 A97 A96 A95 A94 A93 A92 A91 A90 A89 A88 A87 A86 A85 A84 A83 A82 A81 A80 A79 A78 A77 A76 A75 A74 A73 A72 A71 A70 A69 A68 A67 A66 A65 A64 | A135 A134 A133 A132 A131 A130 A129 A128 A127 A126 A125 A124 A123 A122 A121 A120 A119 A118 A117 A116 | A167 A166 A165 A164 A163 A162 A161 A160 A159 A158 A157 A156 L40 L39 L38 L37 A155 A154 A153 A152 A151 A150 A149 A148 A147 A146 A145 A144 L36 L35 L34 L33 A143 A142 A141 A140 A139 A138 A137 A136 | A199 A198 A197 A196 A195 A194 A193 A192 A191 A190 A189 A188 A187 A186 A185 A184 L48 L47 L46 L45 A183 A182 A181 A180 A179 A178 A177 A176 L44 L43 L42 L41 A175 A174 A173 A172 A171 A170 A169 A168 | A251 A250 A249 A248 A247 A246 A245 A244 A243 A242 A241 A240 A239 A238 A237 A236 A235 A234 A233 A232 A231 A230 A229 A228 A227 A226 A225 A224 A223 A222 A221 A220 A219 A218 A217 A216 A215 A214 A213 A212 A211 A210 A209 A208 A207 A206 A205 A204 A203 A202 A201 A200 | A271 A270 A269 A268 A267 A266 A265 A264 A263 A262 A261 A260 A259 A258 A257 A256 A255 A254 A253 A252 | A279 | A281 L60 A280 L57 | A284 L62 A283 L58 | A282 L61 A285 L59 | A286 | A288 L66 A287 L63 | A291 L68 A290 L64 | A289 L67 A292 L65 | A293 | A295 L70 A294 L69 | A299 L73 A298 L71 | A296 L72 A297 L74 | A300 | A302 L76 A301 L75 | A306 L79 A305 L77 | A303 L78 A304 L80 | A307 | A309 L85 A308 L82 | A312 L87 A311 L83 | A310 L86 A313 L84 | A314 | A316 L93 A315 L90 | A319 L95 A318 L91 | A317 L94 A320 L92 | L96 A322 L99 A323 | L97 A324 L100 A325 | L98 A327 L101 A326 | A321 | L102 A328 L105 A333 | L103 A332 L106 A331 | L104 A330 L107 A329 | A334 | A340 L111 A335 L108 | A338 L112 A339 L109 | A336 L113 A337 L110 | A341 | S0 S1 S2 S3 S4 S5 S6 L114 L115 S7 S8 S9 S10 S11 | S19 S20 S21 S22 S23 S24 S25 L116 L117 S26 S27 S28 S29 S30 bodies 2
sketch "Sketch18" plane through (0, 0, -0.2) normal (0, 0, -1) x (-1, 0, 0)
  line L0 (0, 0) -> (-63.5, 0)
  line L1 (-63.5, 0) -> (-63.5, 88.9)
  line L2 (-63.5, 88.9) -> (0, 88.9)
  line L3 (0, 88.9) -> (0, 0)
  constraints: 8 end point, 2 parallel, 1 horizontal, 1 perpendicular
extrude "Extrusion21" add sketch "Sketch18" along normal blind 0.4 bodies 3
fillet "Fillet2" radius 3.175 8 edges at (63.5, 0, 0.2) (63.5, 88.9, 0.2) (0, 0, 0.2) (0, 88.9, 0.2) (63.5, 0, -0.3) (63.5, 88.9, -0.3) (0, 0, -0.3) (0, 88.9, -0.3)
extrude "Extrusion22" cut sketch "Sketch17" along normal blind 0.4 contours A31 A30 A29 A28 A27 A26 A25 A24 A23 A22 A21 A20 L24 L23 L22 L21 A19 A18 A17 A16 A15 A14 A13 A12 A11 A10 A9 A8 L20 L19 L18 L17 A7 A6 A5 A4 A3 A2 A1 A0 | A63 A62 A61 A60 A59 A58 A57 A56 A55 A54 A53 A52 A51 A50 A49 A48 L32 L31 L30 L29 A47 A46 A45 A44 A43 A42 A41 A40 L28 L27 L26 L25 A39 A38 A37 A36 A35 A34 A33 A32 | A115 A114 A113 A112 A111 A110 A109 A108 A107 A106 A105 A104 A103 A102 A101 A100 A99 A98 A97 A96 A95 A94 A93 A92 A91 A90 A89 A88 A87 A86 A85 A84 A83 A82 A81 A80 A79 A78 A77 A76 A75 A74 A73 A72 A71 A70 A69 A68 A67 A66 A65 A64 | A135 A134 A133 A132 A131 A130 A129 A128 A127 A126 A125 A124 A123 A122 A121 A120 A119 A118 A117 A116 | A167 A166 A165 A164 A163 A162 A161 A160 A159 A158 A157 A156 L40 L39 L38 L37 A155 A154 A153 A152 A151 A150 A149 A148 A147 A146 A145 A144 L36 L35 L34 L33 A143 A142 A141 A140 A139 A138 A137 A136 | A199 A198 A197 A196 A195 A194 A193 A192 A191 A190 A189 A188 A187 A186 A185 A184 L48 L47 L46 L45 A183 A182 A181 A180 A179 A178 A177 A176 L44 L43 L42 L41 A175 A174 A173 A172 A171 A170 A169 A168 | A251 A250 A249 A248 A247 A246 A245 A244 A243 A242 A241 A240 A239 A238 A237 A236 A235 A234 A233 A232 A231 A230 A229 A228 A227 A226 A225 A224 A223 A222 A221 A220 A219 A218 A217 A216 A215 A214 A213 A212 A211 A210 A209 A208 A207 A206 A205 A204 A203 A202 A201 A200 | A271 A270 A269 A268 A267 A266 A265 A264 A263 A262 A261 A260 A259 A258 A257 A256 A255 A254 A253 A252 | A279 | A281 L60 A280 L57 | A284 L62 A283 L58 | A282 L61 A285 L59 | A286 | A288 L66 A287 L63 | A291 L68 A290 L64 | A289 L67 A292 L65 | A293 | A295 L70 A294 L69 | A299 L73 A298 L71 | A296 L72 A297 L74 | A300 | A302 L76 A301 L75 | A306 L79 A305 L77 | A303 L78 A304 L80 | A307 | A309 L85 A308 L82 | A312 L87 A311 L83 | A310 L86 A313 L84 | A314 | A316 L93 A315 L90 | A319 L95 A318 L91 | A317 L94 A320 L92 | L96 A322 L99 A323 | L97 A324 L100 A325 | L98 A327 L101 A326 | A321 | L102 A328 L105 A333 | L103 A332 L106 A331 | L104 A330 L107 A329 | A334 | A340 L111 A335 L108 | A338 L112 A339 L109 | A336 L113 A337 L110 | A341 | S0 S1 S2 S3 S4 S5 S6 L114 L115 S7 S8 S9 S10 S11 | S19 S20 S21 S22 S23 S24 S25 L116 L117 S26 S27 S28 S29 S30 bodies 3
